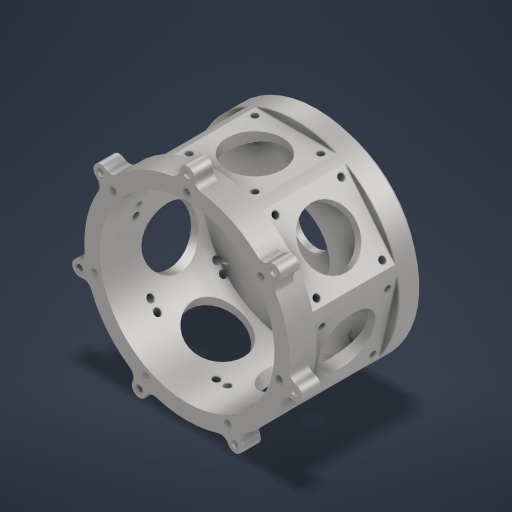
# Autodesk Inventor part: Main Block
Saved by Autodesk Inventor 2023 (Build 270158000, 158)
## iProperties
Created: 2025-05-22
Part Number: Main Block
Material: Generic
Document SubType Name: Modeling
Designer: ryzen
Density: 1 g/cm^3
Appearance: Default
Author: ryzen
Autodesk Inventor part; units mm, degrees
ref_plane "YZ Plane" through (0, 0, 0) normal (1, 0, 0) x (0, 1, 0)
ref_plane "XZ Plane" through (0, 0, 0) normal (0, 1, 0) x (-1, 0, 0)
ref_plane "XY Plane" through (0, 0, 0) normal (0, 0, 1) x (1, 0, 0)
sketch "Sketch1" plane through (0, 0, 0) normal (0, 0, 1) x (1, 0, 0)
  circle A0 centre (0, 0) radius 50
  circle A1 centre (0, 0) radius 45
  circle A2 centre (0, 0) radius 40
  dimension "d0" = 100
  dimension "d1" = 90
  dimension "d2" = 80
  constraints: 3 centre point, 3 coincident
  measures "d0" diameter of A0
  measures "d1" diameter of A1
  measures "d2" diameter of A2
extrude "Extrusion1" add sketch "Sketch1" along normal blind 67 contours A0 | A1 | A2
extrude "Extrusion2" cut sketch "Sketch1" along normal blind 4.07 contours A0
sketch "Sketch2" plane through (0, 0, 67) normal (0, 0, 1) x (1, 0, 0)
  circle A0 centre (0, 0) radius 42.5
  dimension "d7" = 85
  constraints: 1 centre point, 1 coincident
  measures "d7" diameter of A0
extrude "Extrusion3" cut sketch "Sketch2" against normal blind 50
extrude "Extrusion4" cut sketch "Sketch1" along normal blind 13 contours A2
sketch "Sketch3" plane through (0, 0, 13) normal (0, 0, -1) x (-1, 0, 0)
  arc A0 (-8.8696, -23.4732) -> (8.8696, -23.4732) centre (0, -25) ccw
  line L0 (0, -70) -> (0, 70) projected
  arc A1 (11.1939, -18.3561) -> (8.8696, -23.4732) centre (13.7971, -22.625) ccw
  arc A2 (-8.8696, -23.4732) -> (-11.1939, -18.3561) centre (-13.7971, -22.625) ccw
  circle A3 centre (0, -25) radius 4
  arc A4 (24.7632, 4.0554) -> (15.8936, 19.4179) centre (21.6506, 12.5) ccw
  circle A5 centre (21.6506, 12.5) radius 4
  arc A6 (10.2999, 18.8722) -> (15.8936, 19.4179) centre (12.6953, 23.2611) ccw
  arc A7 (24.7632, 4.0554) -> (21.4938, -0.5161) centre (26.4924, -0.6361) ccw
  arc A8 (-15.8936, 19.4179) -> (-24.7632, 4.0554) centre (-21.6506, 12.5) ccw
  circle A9 centre (-21.6506, 12.5) radius 4
  arc A10 (-21.4938, -0.5161) -> (-24.7632, 4.0554) centre (-26.4924, -0.6361) ccw
  arc A11 (-15.8936, 19.4179) -> (-10.2999, 18.8722) centre (-12.6953, 23.2611) ccw
  arc A12 (11.1939, -18.3561) -> (21.4938, -0.5161) centre (0, 0) ccw
  arc A13 (10.2999, 18.8722) -> (-10.2999, 18.8722) centre (0, 0) ccw
  arc A14 (-21.4938, -0.5161) -> (-11.1939, -18.3561) centre (0, 0) ccw
  dimension "d13" = 18
  dimension "d14" = 25
  dimension "d15" = 10
  dimension "d16" = 8
  dimension "d19" = 360
  constraints: 24 point on circle, 15 centre point, 4 coincident, 1 point on line, 1 symmetric about line, 1 tangent, 38 other
  measures "d13" diameter of A0
  measures "d14" distance of point (0, 0) A0.centre
  measures "d15" diameter of A1
  measures "d16" diameter of A3
extrude "Extrusion5" add sketch "Sketch3" along normal blind 9 contours A2 A14 A10 A8 A11 A13 L0 A3 A0 | L0 A3 A13 A6 A4 A7 A12 A1 A0
move or copy body "Rotate1" bodies to move or copy 1 copy no rotation origin (0, 0, 0) rotation axis (0, 0, 1) rotation angle -90
sketch "Sketch4" plane through (0, 0, 17) normal (0, 0, 1) x (1, 0, 0)
  circle A0 centre (0, 0) radius 17.5
  dimension "d25" = 35
  constraints: 1 centre point, 1 coincident
  measures "d25" diameter of A0
extrude "Extrusion6" cut sketch "Sketch4" against normal blind 10
sketch "Sketch5" plane through (0, 0, 7) normal (0, 0, 1) x (1, 0, 0)
  circle A0 centre (0, 0) radius 8.675
  dimension "d28" = 17.35
  constraints: 1 centre point, 1 coincident
  measures "d28" diameter of A0
extrude "Extrusion7" cut sketch "Sketch5" against normal blind 10
chamfer "Chamfer1" distance 2 angle 45 1 edges at (-17.5, 0, 17)
sketch "Sketch6" plane through (0, 0, 0) normal (1, 0, 0) x (0, 1, 0)
  line L0 (45, 4.07) -> (45, 0) projected
  line L1 (45, 0) -> (40, 0) projected
  line L2 (40, 0) -> (40, 13) projected
  line L3 (40, 13) -> (21.533, 13) projected
  line L4 (21.533, 13) -> (21.533, 4) projected
  line L5 (21.533, 4) -> (8.675, 4) projected
  line L6 (8.675, 4) -> (8.675, 7) projected
  line L7 (8.675, 7) -> (17.5, 7) projected
  line L8 (17.5, 7) -> (17.5, 15) projected
  line L9 (17.5, 15) -> (19.5, 17) projected
  line L10 (19.5, 17) -> (42.5, 17) projected
  line L11 (42.5, 17) -> (42.5, 67) projected
  line L12 (42.5, 67) -> (50, 67) projected
  line L13 (50, 67) -> (50, 4.07) projected
  line L14 (50, 4.07) -> (45, 4.07) projected
  line L15 (-45, 0) -> (-45, 4.07) projected
  line L16 (-45, 4.07) -> (-50, 4.07) projected
  line L17 (-50, 4.07) -> (-50, 67) projected
  line L18 (-50, 67) -> (-42.5, 67) projected
  line L19 (-42.5, 67) -> (-42.5, 17) projected
  line L20 (-42.5, 17) -> (-19.5, 17) projected
  line L21 (-19.5, 17) -> (-17.5, 15) projected
  line L22 (-17.5, 15) -> (-17.5, 7) projected
  line L23 (-17.5, 7) -> (-8.675, 7) projected
  line L24 (-8.675, 7) -> (-8.675, 4) projected
  line L25 (-8.675, 4) -> (-21.533, 4) projected
  line L26 (-21.533, 4) -> (-21.533, 13) projected
  line L27 (-21.533, 13) -> (-40, 13) projected
  line L28 (-40, 13) -> (-40, 0) projected
  line L29 (-40, 0) -> (-45, 0) projected
  line L30 (50, 4.07) -> (50, 67) projected
  line L31 (50, 54.07) -> (46, 54.07)
  line L32 (46, 54.07) -> (46, 14.07)
  line L33 (46, 14.07) -> (50, 14.07)
  line L34 (50, 14.07) -> (50, 54.07)
  point P0 (0, 0)
  dimension "d35" = 40
  dimension "d36" = 10
  dimension "d37" = 46
  constraints: 8 end point, 2 parallel, 1 horizontal, 1 perpendicular, 1 point on line
  measures "d35" distance of L33.end L31.start
  measures "d36" distance between parallel lines of L14 L33
  measures "d37" distance from line of point (0, 0) L32
extrude "Extrusion8" cut sketch "Sketch6" along normal mid plane 39.1 contours L33 L32 L31 L13
sketch "Sketch7" plane through (-19.55, 46, 14.07) normal (0, 1, 0) x (1, 0, 0)
  circle A0 centre (19.55, -20) radius 13.5
  line L0 (0, -40) -> (39.1, -40) projected
  line L1 (39.1, 0) -> (0, 0) projected
  line L2 (0, 0) -> (10.1133, -10.3461)
  line L3 (28.9867, -29.6539) -> (39.1, -40)
  line L4 (0, -40) -> (10.1133, -29.6539)
  line L5 (28.9867, -10.3461) -> (39.1, 0)
  line L6 (35.55, -36) -> (3.55, -36)
  line L7 (3.55, -36) -> (3.55, -4)
  line L8 (3.55, -4) -> (35.55, -4)
  line L9 (35.55, -4) -> (35.55, -36)
  line L10 (35.55, -36) -> (3.55, -4) construction
  line L11 (3.55, -36) -> (35.55, -4) construction
  point P0 (19.55, 14.07)
  dimension "d40" = 27
  dimension "d43" = 32
  dimension "d44" = 32
  constraints: 20 end point, 4 point on circle, 2 midpoint, 2 parallel, 1 centre point, 1 coincident, 1 horizontal, 1 perpendicular
  measures "d40" diameter of A0
  measures "d43" distance of L7.end L8.end
  measures "d44" distance of L6.end L7.end
extrude "Extrusion9" cut sketch "Sketch7" against normal blind 39.1 contours A0
hole "Hole2" at (-16, 46, 50.07) at (-16, 46, 18.07) at (16, 46, 18.07) at (16, 46, 50.07) direction (0, -1, 0) diameter 3.242 depth 11.8 tip angle 118 thread size "M4x0.7" class "6H" standard "ISO Metric profile"
sketch "Sketch8" plane through (0, 0, 67) normal (0, 0, 1) x (1, 0, 0)
  circle A0 centre (0, 0) radius 57.275
  arc A1 (3.6365, 53.5518) -> (-3.6365, 53.5518) centre (0, 53.6375) ccw
  circle A2 centre (0, 0) radius 50 projected
  arc A3 (-7.0698, 49.4977) -> (-3.6365, 53.5518) centre (-7.6354, 53.4575) ccw
  arc A4 (3.6365, 53.5518) -> (7.0698, 49.4977) centre (7.6354, 53.4575) ccw
  arc A5 (7.0698, 49.4977) -> (-7.0698, 49.4977) centre (0, 0) ccw
  dimension "d59" = 114.55
  dimension "d61" = 8
  constraints: 10 point on circle, 5 centre point, 4 tangent, 1 coincident, 1 concentric
  measures "d59" diameter of A0
  measures "d61" diameter of A3
extrude "Extrusion10" add sketch "Sketch8" against normal blind 9 contours A1 A4 A2 A3
sketch "Sketch9" plane through (0, 0, 58) normal (0, 0, -1) x (-1, 0, 0)
  arc A0 (3.6365, 53.5518) -> (-3.6365, 53.5518) centre (0, 53.6375) ccw projected
  point P0 (0, 0)
  constraints: 1 coincident
hole "Hole3" at (0, 53.6375, 58) direction (0, 0, 1) diameter 3.4587 depth 11.8 tip angle 118 thread size "M4x0.5" class "6H" standard "ISO Metric profile"
sketch "Sketch10" plane through (0, 53.6375, 67) normal (0, 0, 1) x (1, 0, 0)
  point P0 (0, -53.6375)
  point P1 (0, -7.6375)
  dimension "d71" = 46
  measures "d71" distance of point (0, -53.637) point (0, -7.637)
hole "Hole4" at (0, 46, 67) direction (0, 0, -1) diameter 3.4587 depth 10.8 tip angle 118 thread size "M4x0.5" class "6H" standard "ISO Metric profile"
pattern_circular "Circular Pattern1" count 7 over 360 about axis through (0, 0, 67) along (0, 0, -1) of "Hole4", "Hole3", "Extrusion10", "Hole2", "Extrusion9", "Extrusion8"
sketch "Sketch12" plane through (0, 0, 0) normal (0, 0, -1) x (-1, 0, 0)
  circle A0 centre (0, 0) radius 42.5
  circle A1 centre (0, 0) radius 42.5 projected
  point P0 (0, -42.5)
  dimension "d90" = 85
  constraints: 1 centre point, 1 coincident, 1 vertical alignment, 1 other
  measures "d90" diameter of A0
hole "Hole6" at (0, -42.5, 0) direction (0, 0, 1) diameter 3.4587 depth 10.8 tip angle 118 thread size "M4x0.5" class "6H" standard "ISO Metric profile"
pattern_circular "Circular Pattern2" count 7 over 360 about axis through (0, 0, 67) along (0, 0, -1) of "Hole6"
body "Solid1"
